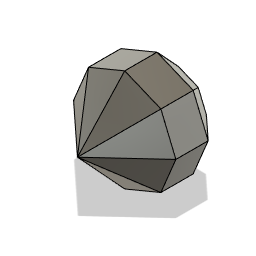
mustem3dmodel (Autodesk Fusion 360 design; units mm, degrees)
Autodesk Fusion 360 part; units mm, degrees
sketch "Sketch1" plane through (0, 0, 0) normal (0, 0, 1) x (1, 0, 0)
  line L0 (0, 95) -> (-67.1751, 67.1751)
  line L1 (-67.1751, 67.1751) -> (-95, 0)
  line L2 (-95, 0) -> (-67.1751, -67.1751)
  line L3 (-67.1751, -67.1751) -> (0, -95)
  line L4 (0, -95) -> (67.1751, -67.1751)
  line L5 (67.1751, -67.1751) -> (95, 0)
  line L6 (95, 0) -> (67.1751, 67.1751)
  line L7 (67.1751, 67.1751) -> (0, 95)
  dimension "d6" = 95
  dimension "d16" = 72.7099
  measures "d6" distance of L0.start origin
  measures "d16" distance of L0.start L6.end
extrude "Extrude2" add sketch "Sketch1" along normal blind 100 draft -45
shell "Shell2" thickness 3 removed faces 1 at (-22.3917, 22.3917, 0)
sketch "Sketch3" plane through (0, 0, 0) normal (0, 0, 1) x (1, 0, 0)
  line L0 (0, 95) -> (-67.1751, 67.1751)
  line L1 (-67.1751, 67.1751) -> (-95, 0)
  line L2 (-95, 0) -> (-67.1751, -67.1751)
  line L3 (-67.1751, -67.1751) -> (0, -95)
  line L4 (0, -95) -> (67.1751, -67.1751)
  line L5 (67.1751, -67.1751) -> (95, 0)
  line L6 (95, 0) -> (67.1751, 67.1751)
  line L7 (67.1751, 67.1751) -> (0, 95)
  line L8 (0, -90.3998) -> (63.9223, -63.9223)
  line L9 (63.9223, -63.9223) -> (90.3998, 0)
  line L10 (90.3998, 0) -> (63.9223, 63.9223)
  line L11 (63.9223, 63.9223) -> (0, 90.3998)
  line L12 (0, 90.3998) -> (-63.9223, 63.9223)
  line L13 (-63.9223, 63.9223) -> (-90.3998, 0)
  line L14 (-90.3998, 0) -> (-63.9223, -63.9223)
  line L15 (-63.9223, -63.9223) -> (0, -90.3998)
  dimension "d22" = -4.25
extrude "Extrude3" add sketch "Sketch3" against normal blind 60
sketch "Sketch4" plane through (0, 0, -60) normal (0, 0, -1) x (-1, 0, 0)
  line L0 (95, 0) -> (67.1751, 67.1751)
  line L1 (67.1751, 67.1751) -> (0, 95)
  line L2 (0, 95) -> (-67.1751, 67.1751)
  line L3 (-67.1751, 67.1751) -> (-95, 0)
  line L4 (-95, 0) -> (-67.1751, -67.1751)
  line L5 (-67.1751, -67.1751) -> (0, -95)
  line L6 (0, -95) -> (67.1751, -67.1751)
  line L7 (67.1751, -67.1751) -> (95, 0)
  line L8 (0, 90.3998) -> (-63.9223, 63.9223)
  line L9 (-63.9223, 63.9223) -> (-90.3998, 0)
  line L10 (-90.3998, 0) -> (-63.9223, -63.9223)
  line L11 (-63.9223, -63.9223) -> (0, -90.3998)
  line L12 (0, -90.3998) -> (63.9223, -63.9223)
  line L13 (63.9223, -63.9223) -> (90.3998, 0)
  line L14 (90.3998, 0) -> (63.9223, 63.9223)
  line L15 (63.9223, 63.9223) -> (0, 90.3998)
  dimension "d23" = -4.25
extrude "Extrude4" add sketch "Sketch4" along normal blind 40 draft -45 contours L0 L1 L2 L3 L4 L5 L6 L7 | L8 L9 L10 L11 L12 L13 L14 L15
sketch "Sketch5" plane through (-40.5438, -16.7938, 43.8843) normal (-0.653281, -0.270598, 0.707107) x (0.73451, 0, 0.678598)
  line L0 (-49.3408, -52.3338) -> (59.5596, 17.4446)
  line L1 (59.5596, 17.4446) -> (-69.7784, 17.4446)
  circle A0 centre (-8.8575, -0.7386) radius 4.1
  line L2 (-69.7784, 17.4446) -> (-49.3408, -52.3338)
  dimension "d17" = 8.2
  measures "d17" diameter of A0
extrude "Extrude5" cut sketch "Sketch5" against normal blind 5 contours A0
sketch "Sketch6" plane through (-33.5876, -81.0876, 0) normal (-0.382683, -0.92388, 0) x (0, 0, 1)
  line L0 (0, -27.6541) -> (0, 34.312)
  line L1 (0, 34.4447) -> (-60, 34.4447)
  line L2 (-60, 34.4447) -> (-60, -34.4447)
  line L3 (-60, -34.4447) -> (0, -34.4447)
  line L4 (0, 34.312) -> (0, 34.4447)
  line L5 (-51.5, 28.9527) -> (-8.5, 28.9527)
  line L6 (-8.5, 28.9527) -> (-8.5, -31.3473)
  line L7 (-8.5, -31.3473) -> (-51.5, -31.3473)
  line L8 (-51.5, -31.3473) -> (-51.5, 28.9527)
  line L9 (0, -34.4447) -> (0, -27.6541)
  line L10 (0, -37.5473) -> (-60, -37.5473)
  line L11 (0, -36.3549) -> (0, 36.3549)
  line L12 (0, 36.3549) -> (-60, 36.3549)
  line L13 (-60, 36.3549) -> (-60, -36.3549)
  line L14 (-60, -36.3549) -> (0, -36.3549)
  dimension "d20" = 43
  dimension "d21" = 60.3
  dimension "d24" = 8.5
  dimension "d25" = 6.2
  constraint horizontal L5
  constraint vertical L6
  constraint horizontal L7
  constraint vertical L8
  measures "d20" distance of L5.start L5.end
  measures "d21" distance of L5.start L7.end
  measures "d24" distance of L2 L8
  measures "d25" distance of L7 L10
extrude "Extrude6" cut sketch "Sketch6" against normal blind 5 contours L5 L6 L7 L8
